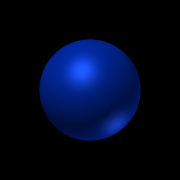
# Autodesk Inventor part: Ball
Saved by Autodesk Inventor 2012 (Build 160160000, 160)
## iProperties
Created: 2012-10-02
Part Number: Ball
Material: Rubber
Document SubType Name: Modeling
Designer: agmlego
Density: 0.93 g/cm^3
Mass: 22.1475 g
Surface Area: 187.786 cm^2
Volume: 23.8145 cm^3
Author: agmlego
Autodesk Inventor part; units mm, degrees
ref_plane "YZ Plane" through (0, 0, 0) normal (1, 0, 0) x (0, 1, 0)
ref_plane "XZ Plane" through (0, 0, 0) normal (0, 1, 0) x (-1, 0, 0)
ref_plane "XY Plane" through (0, 0, 0) normal (0, 0, 1) x (1, 0, 0)
sketch "Sketch2" plane through (0, 0, 0) normal (0, 0, 1) x (1, 0, 0)
  arc A0 (28.575, 0) -> (-28.575, 0) centre (0, 0) ccw
  line L0 (-28.575, 0) -> (-28.575, -70.3192) construction
  line L1 (28.575, 0) -> (28.575, -70.3192) construction
  arc A1 (26.035, 0) -> (-26.035, 0) centre (0, 0) ccw
  line L2 (-28.575, 0) -> (-26.035, 0)
  line L3 (26.035, 0) -> (28.575, 0)
  dimension "d0" = 28.575
  dimension "d3" = 2.54
  constraints: 8 end point, 4 point on circle, 2 centre point, 2 coincident, 2 horizontal, 2 perpendicular, 2 tangent, 1 parallel
  measures "d0" radius of A0
  measures "d3" radial gap between concentric circles of A0 A1
revolve "Revolution2" add sketch "Sketch2" angle 360 about axis through (-28.575, 0, 0) along (1, 0, 0)
body "Solid2"
